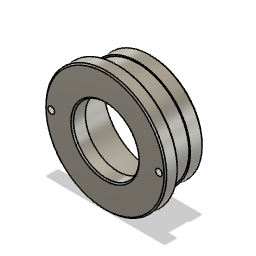
cryo head flange v5 (Autodesk Fusion 360 design; units mm, degrees)
Autodesk Fusion 360 part; units mm, degrees
sketch "Sketch2" plane through (0, 0, 0) normal (0, 0, 1) x (1, 0, 0)
  circle A0 centre (0, 0) radius 46
  circle A1 centre (0, 0) radius 25
  line L0 (0, 1.75) -> (0, 22.5) construction
  circle A2 centre (0, 0) radius 36
  point P0 (-41, 0)
  point P1 (41, 0)
  dimension "d4" = 50
  dimension "d5" = 82
  dimension "d6" = 92
  dimension "d7" = -10
  constraint horizontal A0.centre P0
  constraint horizontal A0.centre P1
  constraint coincident A0.centre A1.centre
  constraint symmetric P0 P1 L0
  measures "d4" diameter of A1
  measures "d5" distance of P0 P1
  measures "d6" diameter of A0
extrude "Extrude1" add sketch "Sketch2" against normal blind 35 contours A0
extrude "Extrude2" add sketch "Sketch2" against normal blind 10 contours A2
hole "Hole1" at (-41, 0, 0) at (41, 0, 0) direction (0, 0, -1) diameter 5.035 depth 10 tip angle 118
thread "Thread1" "ISO Metric profile 6.0 M6x1 6H" thread offset 0 thread depth 10
sketch "Sketch3" plane through (0, 0, 0) normal (1, 0, 0) x (0, 0, -1)
  line L0 (10, 46) -> (10, 39)
  line L1 (10, 39) -> (25, 39)
  line L2 (25, 39) -> (25, 40)
  line L3 (25, 40) -> (35, 40)
  line L4 (-1.75, 0) -> (-22.5, 0) construction
  line L5 (35, -46) -> (35, 46)
  line L6 (0, 46) -> (0, -46)
  line L7 (35, 46) -> (10, 46)
  dimension "d15" = 40
  dimension "d16" = 1
  dimension "d17" = 25
  dimension "d18" = 10
  constraint vertical L0
  constraint perpendicular L0 L1
  constraint perpendicular L1 L2
  constraint perpendicular L0 L3
  constraint coincident L5.end L7.start
  constraint coincident L0 L7.end
  constraint perpendicular L0 L7
  constraint coincident L3.end L5
  measures "d15" distance of L3 L4
  measures "d16" distance of L1 L3
  measures "d17" distance of L0 L5
  measures "d18" distance of L2.end L3.end
revolve "Revolve1" cut sketch "Sketch3" angle 360 about axis through (0, 0, 1.75) along (0, 0, 1)
chamfer "Chamfer1" distance 1 angle 45 4 edges at (-42.8871, -16.6343, 0) (-42.8871, -16.6343, -10) (-14.4646, -37.2931, -35) (-23.3082, 9.0404, 0)
